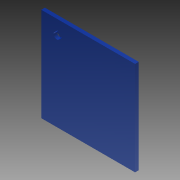
# Autodesk Inventor part: tray
Saved by Autodesk Inventor 2014 SP2 (Build 180246200, 246)
## iProperties
Created: 2016-04-26
Part Number: tray
Material: Generic
Document SubType Name: Modeling
Designer: cruiser
Density: 1 g/cm^3
Appearance: Clear - Blue
Author: cruiser
Autodesk Inventor part; units mm, degrees
ref_plane "YZ Plane" through (0, 0, 0) normal (1, 0, 0) x (0, 1, 0)
ref_plane "XZ Plane" through (0, 0, 0) normal (0, 1, 0) x (-1, 0, 0)
ref_plane "XY Plane" through (0, 0, 0) normal (0, 0, 1) x (1, 0, 0)
sketch "Sketch1" plane through (0, 0, 0) normal (0, 1, 0) x (-1, 0, 0)
  line L0 (75.5, -75.5) -> (-75.5, -75.5)
  line L1 (-75.5, -75.5) -> (-75.5, 75.5)
  line L2 (-75.5, 75.5) -> (75.5, 75.5)
  line L3 (75.5, 75.5) -> (75.5, -75.5)
  line L4 (75.5, -75.5) -> (-75.5, 75.5) construction
  line L5 (-75.5, -75.5) -> (75.5, 75.5) construction
  point P0 (0, 0)
  dimension "d0" = 151
  dimension "d1" = 151
  constraints: 12 end point, 2 midpoint, 2 parallel, 1 horizontal, 1 perpendicular
  measures "d0" distance of L1.end L2.end
  measures "d1" distance of L0.end L1.end
extrude "Extrusion1" add sketch "Sketch1" along normal blind 5.88
sketch "Sketch2" plane through (0, 5.88, 0) normal (0, 1, 0) x (1, 0, 0)
  circle A0 centre (-50.6605, -51.576) radius 5
  point P0 (0, 0)
  dimension "d4" = 10
  constraints: 1 centre point
  measures "d4" diameter of A0
extrude "Extrusion2" cut sketch "Sketch2" against normal blind 5.88
equation "\"d0\" = reservoir_x"
equation "\"d1\" = reservoir_y"
equation "\"d2\" = thick_acrylic"
equation "\"d4\" = stopper_diameter"
equation "\"d5\" = thick_acrylic"
equation "\"sm_thickness\" = 1.5875"
equation "\"thick_acrylic\" = 5.88"
equation "\"thin_acrylic\" = 3.15"
equation "\"clear_acrylic\" = 3.15"
equation "\"wood_thickness\" = 6.72"
equation "\"m3_diameter\" = 3.15"
equation "\"m4_diameter\" = 4.2"
equation "\"m5_diameter\" = 5.25"
equation "\"brass_insert_drill\" = 4"
equation "\"m5_brass_insert_drill\" = 6.7"
equation "\"m3_main_length\" = 14"
equation "\"m3_main_nut_width\" = 5.7"
equation "\"m3_main_nut_thickness\" = 2.5"
equation "\"m3_main_extra\" = 1"
equation "\"stepper_screw_space\" = 35"
equation "\"stepper_shaft_diameter\" = 5"
equation "\"stepper_body_diameter\" = 28"
equation "\"laser_body_diameter\" = 12"
equation "\"t_carrier\" = 5.88"
equation "\"t_wall\" = 5.88"
equation "\"t_window\" = 3.15"
equation "\"carrier_y\" = 181"
equation "\"carrier_z\" = 12"
equation "\"carrier_z2\" = 283.04"
equation "\"protection_slot\" = 36.2"
equation "\"protection_slot_offset\" = 45.25"
equation "\"protection_slot_length\" = 35"
equation "\"window_z\" = 185"
equation "\"window_y\" = 49.56"
equation "\"window_slot\" = 25"
equation "\"door_sensor\" = 35"
equation "\"reservoir_x\" = 151"
equation "\"reservoir_y\" = 151"
equation "\"reservoir_z\" = 25.4"
equation "\"reservoir_overlap\" = 5"
equation "\"linear_bearing_spacing\" = 207"
equation "\"linear_bearing_z\" = 304.8"
equation "\"threaded_rod_z\" = 203.2"
equation "\"motor_spacing\" = 287"
equation "\"t_tray\" = 3.15"
equation "\"tray_border\" = 15"
equation "\"tray_x\" = 181"
equation "\"tray_y\" = 181"
equation "\"bed_x\" = 141"
equation "\"bed_y\" = 141"
equation "\"stopper_diameter\" = 10"
equation "\"brass_keep_out\" = 8"
equation "\"tape_keep_out\" = 2"
equation "\"tape_thickness\" = 2"
equation "\"t_crane\" = 6.72"
equation "\"crane_x\" = 258"
equation "\"crane_z\" = 45"
equation "\"end_stop_offset_x\" = 47"
equation "\"end_stop_spacing\" = 19"
equation "\"thumb_nut_offset_y\" = 11.72"
equation "\"thumb_nut_diameter\" = 7"
equation "\"z_min_from_center\" = 79"
equation "\"t_frame\" = 6.72"
equation "\"frame_top_z\" = 291"
equation "\"frame_bottom_z\" = 225"
equation "\"frame_total_z\" = 516"
equation "\"frame_y\" = 68.44"
equation "\"frame_border\" = 39.5"
equation "\"frame_foot_z\" = 49.5"
equation "\"frame_tilt\" = 1deg"
equation "\"printer_z\" = 289"
equation "\"lcd_x\" = 72"
equation "\"lcd_y\" = 25"
equation "\"subframe_y_offset\" = 27.5"
equation "\"laser_y_offset\" = 19.4"
equation "\"laser_diameter\" = 12"
equation "\"laser_z_offset\" = 55"
equation "\"laser_y\" = 35"
equation "\"laser_z\" = 18"
equation "\"laser_x\" = 24"
equation "\"t_galvo_frame\" = 6.72"
equation "\"galvo_frame_x\" = 66"
equation "\"galvo_frame_z\" = 65"
equation "\"galvo_frame_y_offset\" = 27.5"
equation "\"drawer_x\" = 187.3"
equation "\"drawer_y\" = 57.8425"
equation "\"drawer_z\" = 206.72"
equation "\"drawer_z_from_bottom\" = 25"
equation "\"crane_z2\" = 12"
equation "\"bed_z\" = 25.4"
equation "\"nema17_x\" = 43"
body "Solid1"
